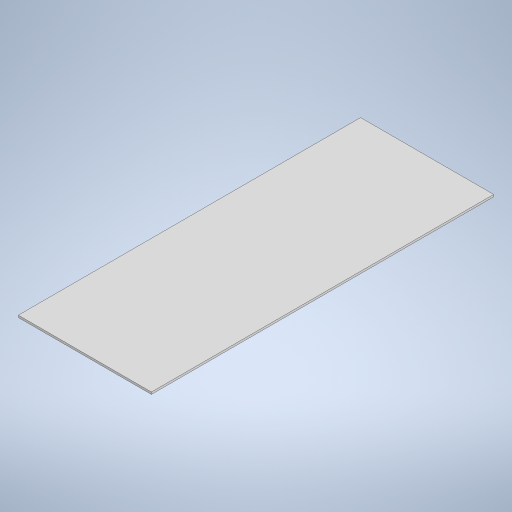
# Autodesk Inventor part: Cheap polycarp
Saved by Autodesk Inventor 2024 (Build 280153000, 153)
## iProperties
Created: 2023-05-31
Part Number: Cheap polycarp
Material: Generic
Document SubType Name: Modeling
Designer: labra
Density: 1 g/cm^3
Appearance: Default
Author: labra
Autodesk Inventor part; units mm, degrees
ref_plane "YZ Plane" through (0, 0, 0) normal (1, 0, 0) x (0, 1, 0)
ref_plane "XZ Plane" through (0, 0, 0) normal (0, 1, 0) x (-1, 0, 0)
ref_plane "XY Plane" through (0, 0, 0) normal (0, 0, 1) x (1, 0, 0)
sketch "Sketch1" plane through (0, 0, 0) normal (0, 1, 0) x (-1, 0, 0)
  line L0 (0, 0) -> (355.6, 0)
  line L1 (355.6, 0) -> (355.6, -914.4)
  line L2 (355.6, -914.4) -> (0, -914.4)
  line L3 (0, -914.4) -> (0, 0)
  point P0 (177.8, -914.4)
  dimension "d0" = 914.4
  dimension "d1" = 355.6
  constraints: 8 end point, 2 parallel, 1 horizontal, 1 midpoint, 1 perpendicular
  measures "d0" distance from line of point (177.8, -914.4) L0
  measures "d1" distance between parallel lines of L3 L1
extrude "Extrusion1" add sketch "Sketch1" along normal blind 5.588
body "Solid1"
